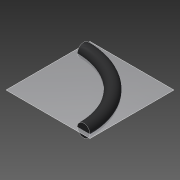
# Autodesk Inventor part: Cable
Saved by Autodesk Inventor 2015 SP1 (Build 190203100, 203)
## iProperties
Created: 2014-11-07
Part Number: Cable
Material: Generic
Document SubType Name: Modeling
Designer: Cody Redding
Density: 1 g/cm^3
Appearance: Rubber - Black
Description: Generic Cable
RuleStatus: InUse
Author: Cody Redding
Autodesk Inventor part; units mm, degrees
note: some values were not read from the file. Chosen so that the rebuilt part matches the saved one: bend side of "Bend Part1".
ref_plane "XY Plane" through (0, 0, 0) normal (0, 0, 1) x (1, 0, 0)
sketch "Sketch2" plane through (0, 0, 0) normal (0, 0, 1) x (1, 0, 0)
  circle A0 centre (0, 0) radius 3.175
  constraints: 1 centre point, 1 coincident, 1 other
extrude "Extrusion1" add sketch "Sketch2" against normal blind 49.8728
ref_plane "Work Plane1" through (-3.175, 0, 0) normal (1, 0, 0) x (0, 1, 0)
sketch "Sketch3" plane through (-3.175, 0, 0) normal (1, 0, 0) x (0, 1, 0)
  line L0 (-3.175, -49.8728) -> (3.175, -49.8728) projected
  line L1 (-3.175, 0) -> (3.175, 0) projected
  point P0 (0, 0)
bend part "Bend Part1" radius 31.75 angle 90 line through (-3.175, -3.175, 0) along (0, 1, 0) centre toward (-1, 0, 0) moving side (0, 0, -1) both sides no
equation "\"d1\" = Arc_Length"
equation "\"Arc_Length\" = 49.87278"
equation "\"Cable_Rad\" = 3.175"
body "Solid1"
